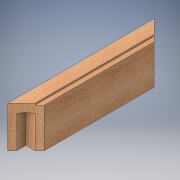
# Autodesk Inventor part: SideWidthOutlet
Saved by Autodesk Inventor 2016 (Build 200138000, 138)
## iProperties
Created: 2016-02-09
Part Number: SideWidthOutlet
Material: Wood (Birch)
Document SubType Name: Modeling
Designer: ron
Density: 0.55 g/cm^3
Appearance: Birch - Natural Polished
Mass: 4851.38 g
Surface Area: 3661.94 cm^2
Volume: 8820.7 cm^3
Author: ron
Autodesk Inventor part; units mm, degrees
ref_plane "YZ Plane" through (0, 0, 0) normal (1, 0, 0) x (0, 1, 0)
ref_plane "XZ Plane" through (0, 0, 0) normal (0, 1, 0) x (-1, 0, 0)
sketch "Sketch1" plane through (0, 0, 0) normal (0, 0, 1) x (1, 0, 0)
  line L0 (0, 0) -> (0, 228.6)
  line L1 (0, 228.6) -> (76.2, 228.6)
  line L2 (76.2, 228.6) -> (76.2, 219.2528)
  line L3 (76.2, 219.2528) -> (101.6, 219.2528)
  line L4 (101.6, 219.2528) -> (101.6, 0)
  line L5 (101.6, 0) -> (0, 0)
  dimension "d0" = 228.6
  dimension "d1" = 76.2
  dimension "d2" = 9.3472
  dimension "d3" = 25.4
  constraints: 12 end point, 5 perpendicular, 1 vertical
  measures "d0" distance of L0.start L0.end
  measures "d1" distance of L0.end L1.end
  measures "d2" distance of L1.end L2.end
  measures "d3" distance of L2.end L3.end
extrude "Extrusion1" add sketch "Sketch1" along normal blind 812.8
sketch "Sketch6" plane through (0, 0, 0) normal (0, -1, 0) x (1, 0, 0)
  line L0 (101.6, 0) -> (101.6, 812.8) projected
  line L1 (0, 812.8) -> (101.6, 711.2) projected
  line L2 (76.2038, 736.5962) -> (25.4038, 736.5962)
  line L3 (25.4038, 736.5962) -> (25.4038, 787.3962)
  line L4 (25.4038, 787.3962) -> (76.2, 736.6)
  point P0 (0, 0)
  point P1 (101.6, 101.6)
  dimension "d31" = 35.9156
  dimension "d32" = 50.8
  dimension "d33" = 50.8
  constraints: 6 end point, 2 point on line, 1 horizontal
  measures "d31" distance of L1.end L2.start
  measures "d32" distance of L2.start L2.end
  measures "d33" distance of L2.end L3.end
extrude "Extrusion4" cut sketch "Sketch6" against normal blind 181.1528
sketch "Sketch7" plane through (25.4038, 0, 736.5962) normal (0, -1, 0) x (1, 0, 0)
  line L0 (76.1962, -634.9962) -> (50.7962, -660.3962)
  line L1 (50.7962, -660.3962) -> (-0.0038, -660.3962)
  line L2 (76.1962, -634.9962) -> (-25.4038, -736.5962) projected
  line L3 (76.1962, -736.5962) -> (76.1962, 76.2038) projected
  line L4 (-0.0038, -660.3962) -> (-0.0038, -711.1962)
  line L5 (-0.0038, -711.1962) -> (50.7962, -660.3962)
  point P0 (76.1962, -25.3962)
  dimension "d39" = 50.8
  dimension "d41" = 90
  dimension "d42" = 50.8
  constraints: 8 end point, 1 collinear, 1 point on line
  measures "d39" distance of L0.end L1.end
  measures "d41" angle of L3 L1
  measures "d42" distance of L1.end L4.end
extrude "Extrusion5" cut sketch "Sketch7" against normal blind 181.1528
chamfer "Chamfer5" distance 101.6 angle 45 1 edges at (101.6, 109.6264, 812.8)
chamfer "Chamfer6" distance 101.6 angle 45 1 edges at (101.6, 109.6264, 0)
ref_plane "Work Plane3" through (137.521, 56.9702, 137.521) normal (0.7071068, 0, 0.7071068) x (0, -1, 0)
sketch "Sketch9" plane through (137.521, 56.9702, 137.521) normal (0.7071068, 0, 0.7071068) x (0, -1, 0)
  line L0 (-162.2826, 0) -> (-162.2826, -466.9733) projected
  line L1 (-162.2826, 0) -> (-48.0842, 0)
  line L2 (-162.2826, 0) -> (56.9702, 0) projected
  dimension "d65" = 114.1984
  constraints: 2 end point, 1 point on line
  measures "d65" distance of L0.start L1.end
hole "Hole2" at (137.521, 105.0544, 137.521) direction (-0.7071068, 0, -0.7071068) diameter 12.7 depth 127 tip angle 118
sketch "Sketch10" plane through (0, 181.1528, 0) normal (0, -1, 0) x (1, 0, 0)
  line L0 (76.2, 76.2) -> (76.2, 736.6) projected
  line L1 (76.2, 76.2) -> (63.5019, 63.5019)
  line L2 (0, 0) -> (76.2, 76.2) projected
  line L3 (63.5019, 63.5019) -> (38.1019, 63.5019)
  line L4 (38.1019, 63.5019) -> (38.1019, 38.1019)
  line L5 (63.5019, 63.5019) -> (38.1019, 38.1019)
  line L6 (76.2038, 736.5962) -> (63.5058, 749.2942)
  line L7 (63.5058, 749.2942) -> (38.1058, 749.2942)
  line L8 (38.1058, 749.2942) -> (38.1058, 774.6942)
  line L9 (63.5058, 749.2942) -> (38.1058, 774.6942)
  dimension "d73" = 17.9578
  dimension "d74" = 25.4
  dimension "d75" = 17.9578
  dimension "d76" = 25.4
  constraints: 16 end point, 2 collinear, 2 horizontal, 2 perpendicular, 2 point on line
  measures "d73" distance of L0.start L1.end
  measures "d74" distance of L1.end L3.end
  measures "d75" distance of L6.start L6.end
  measures "d76" distance of L6.end L7.end
extrude "Extrusion6" cut sketch "Sketch10" against normal blind 3.175 contours L7 L8 L9
sketch "Sketch11" plane through (25.4038, 181.1528, 736.5962) normal (0, -1, 0) x (1, 0, 0)
  line L0 (50.7962, -660.3962) -> (38.0981, -673.0942)
  line L1 (38.0981, -673.0942) -> (12.6962, -673.0942)
  line L2 (12.6962, -673.0942) -> (12.6962, -698.4962)
  line L3 (38.0981, -673.0942) -> (12.6962, -698.4962)
  line L4 (-25.4038, -736.5962) -> (50.7962, -660.3962) projected
  dimension "d79" = 17.9578
  dimension "d80" = 180
  dimension "d81" = 25.4019
  dimension "d82" = 25.4019
  constraints: 8 end point, 1 horizontal
  measures "d79" distance of L0.start L0.end
  measures "d80" angle of L4 L0
  measures "d81" distance of L0.end L1.end
  measures "d82" distance of L1.end L2.end
extrude "Extrusion7" cut sketch "Sketch11" against normal blind 3.175
body "Solid1"
